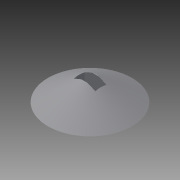
# Autodesk Inventor part: Base
Saved by Autodesk Inventor 2014 (Build 180170000, 170)
## iProperties
Created: 2017-08-29
Part Number: Base
Material: Generic
Document SubType Name: Modeling
Designer: resaj
Density: 1 g/cm^3
Appearance: Default
Author: resaj
Autodesk Inventor part; units mm, degrees
ref_plane "YZ Plane" through (0, 0, 0) normal (1, 0, 0) x (0, 1, 0)
ref_plane "XZ Plane" through (0, 0, 0) normal (0, 1, 0) x (-1, 0, 0)
ref_plane "XY Plane" through (0, 0, 0) normal (0, 0, 1) x (1, 0, 0)
sketch "Sketch1" plane through (0, 0, 0) normal (0, 1, 0) x (-1, 0, 0)
  circle A0 centre (0, 0) radius 20
  dimension "d0" = 40
  constraints: 1 centre point, 1 coincident
  measures "d0" diameter of A0
extrude "Extrusion1" add sketch "Sketch1" along normal blind 10
sketch "Sketch2" plane through (0, 10, 0) normal (0, 1, 0) x (1, 0, 0)
  circle A0 centre (0, 0) radius 20 projected
  line L0 (0, 0) -> (0, 20) construction
  line L1 (0, 0) -> (20, 0) construction
  line L2 (0, 2.65) -> (5.15, 2.65)
  line L3 (5.15, 2.65) -> (5.15, 0)
  line L4 (0, 2.65) -> (-5.15, 2.65)
  line L5 (-5.15, 2.65) -> (-5.15, 0)
  line L6 (0, -2.65) -> (5.15, -2.65)
  line L7 (5.15, -2.65) -> (5.15, 0)
  line L8 (0, -2.65) -> (-5.15, -2.65)
  line L9 (-5.15, -2.65) -> (-5.15, 0)
  dimension "d5" = 5.3
  dimension "d6" = 10.3
  constraints: 20 end point, 5 symmetric about line, 2 perpendicular, 2 point on circle, 2 point on line, 1 parallel, 1 vertical
  measures "d5" distance between parallel lines of L6 L2
  measures "d6" distance between parallel lines of L5 L3
extrude "Extrusion2" cut sketch "Sketch2" against normal through all contours L2 L3 L7 L6 L8 L9 L5 L4
chamfer "Chamfer1" distance 17 distance2 10 1 edges at (20, 10, 0) measured on face at (19.5, 10, 0)
body "Solid1"
